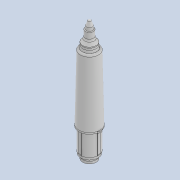
# Autodesk Inventor part: маркер
Saved by Autodesk Inventor 2021.2 (Build 252289000, 289)
## iProperties
Created: 2026-09-22
Part Number: маркер
Material: Типовые
Document SubType Name: Modeling
Designer: ritar
Density: 1 g/cm^3
Appearance: По умолчанию
Author: ritar
Autodesk Inventor part; units mm, degrees
ref_plane "YZ Plane" through (0, 0, 0) normal (1, 0, 0) x (0, 1, 0)
ref_plane "XZ Plane" through (0, 0, 0) normal (0, 1, 0) x (-1, 0, 0)
ref_plane "XY Plane" through (0, 0, 0) normal (0, 0, 1) x (1, 0, 0)
sketch "Эскиз1" plane through (0, 0, 0) normal (0, 0, 1) x (1, 0, 0)
  line L0 (0, 0) -> (-11.15, 0)
  line L1 (-11.15, 0) -> (-9.75, 67.9856)
  line L2 (-9.75, 67.9856) -> (0, 67.9856)
  line L3 (0, 67.9856) -> (0, 0)
  line L4 (0, 67.9856) -> (0, 70.4856)
  line L5 (-9.75, 67.9856) -> (-9.6985, 70.4856)
  line L6 (0, 70.4856) -> (-9.6985, 70.4856)
  dimension "d0" = 11.15
  dimension "d1" = 9.75
  dimension "d2" = 68
  dimension "d3" = 2.5
  constraints: 14 end point, 3 horizontal, 1 collinear, 1 perpendicular, 1 point on line
  measures "d0" distance of L0.start L0.end
  measures "d1" distance of L1.end L2.end
  measures "d2" distance of L0.end L1.end
  measures "d3" distance of L2.end L4.end
revolve "Вращение1" add sketch "Эскиз1" angle 360 about axis through (0, 67.9856, 0) along (0, -1, 0)
fillet "Сопряжение1" radius 2 1 edges at (9.6985, 70.4856, 0)
sketch "Эскиз2" plane through (0, 0, 0) normal (0, 0, 1) x (1, 0, 0)
  line L0 (-7.7393, 70.4856) -> (7.7393, 70.4856) projected
  line L1 (0, 70.4856) -> (0, 72.9856)
  line L2 (0, 72.9856) -> (-7.2, 72.9856)
  line L3 (-7.2, 72.9856) -> (-7.7, 70.4856)
  line L4 (0, 72.9856) -> (-7.2, 72.9856)
  line L5 (-7.2, 72.9856) -> (-7.2, 74.9856)
  line L6 (-7.2, 74.9856) -> (0, 74.9856)
  line L7 (0, 74.9856) -> (0, 72.9856)
  line L8 (-7.2, 75.9856) -> (0, 75.9856)
  line L9 (0, 75.9856) -> (0, 74.9856)
  arc A0 (-7.2, 75.9856) -> (-7.2, 74.9856) centre (-4.725, 75.4856) ccw
  line L10 (-7.2, 75.9856) -> (-4.3, 79.9856)
  line L11 (-4.3, 79.9856) -> (0, 79.9856)
  line L12 (0, 79.9856) -> (0, 75.9856)
  line L13 (-4.3, 79.9856) -> (0, 79.9856)
  line L14 (0, 79.9856) -> (0, 87.4856)
  line L15 (0, 87.4856) -> (-4.3, 87.4856)
  line L16 (-4.3, 87.4856) -> (-4.3, 79.9856)
  arc A1 (-5.025, 78.9856) -> (-4.3, 81.2207) centre (-8.108, 81.2207) ccw
  line L17 (0, 87.4856) -> (-3.075, 87.4856)
  line L18 (-3.075, 87.4856) -> (-3.075, 90.9856)
  line L19 (-3.075, 90.9856) -> (0, 90.9856)
  line L20 (0, 90.9856) -> (0, 87.4856)
  line L21 (-3.075, 90.9856) -> (-1.5669, 95.3677)
  arc A2 (0, 96.4856) -> (-1.5669, 95.3677) centre (0, 94.8285) ccw
  line L22 (0, 90.9856) -> (0, 96.4856)
  point P0 (0, 0)
  point P1 (-7.25, 75.4856)
  point P2 (-3.075, 87.4856)
  dimension "d6" = 7.2
  dimension "d7" = 7.7
  dimension "d8" = 2.5
  dimension "d9" = 2
  dimension "d10" = 1
  dimension "d12" = 0.05
  dimension "d13" = 4.3
  dimension "d14" = 4
  dimension "d15" = 17
  dimension "d16" = 1
  dimension "d17" = 1.2352
  dimension "d18" = 3.075
  dimension "d19" = 3.5
  dimension "d20" = 5.5
  constraints: 44 end point, 7 parallel, 7 point on circle, 5 horizontal, 5 perpendicular, 3 centre point, 3 point on line, 3 tangent, 3 vertical alignment, 2 vertical, 1 midpoint
  measures "d6" distance of L2.end L1.end
  measures "d7" distance from line of L3.end L1
  measures "d8" distance of L1.start L1.end
  measures "d9" distance of L6.end L1.end
  measures "d10" distance of L8.end L6.end
  measures "d12" horizontal distance of L5.end point (-7.25, 75.486)
  measures "d13" distance of L10.end L11.end
  measures "d14" distance of L11.end L8.end
  measures "d15" distance between parallel lines of L0 L15
  measures "d16" distance from line of L11 A1.start
  measures "d17" vertical distance of L11.end A1.end
  measures "d18" distance of L18.end L19.end
  measures "d19" distance of L17.end L18.end
  measures "d20" distance of L19.end L22.end
revolve "Вращение2" add sketch "Эскиз2" angle 360 about axis through (0, 79.9856, 0) along (0, 1, 0)
sketch "Эскиз3" plane through (0, 0, 0) normal (0, -1, 0) x (1, 0, 0)
  circle A0 centre (0, 0) radius 11.15 projected
extrude "Выдавливание1" add sketch "Эскиз3" along normal blind 1.5
sketch "Эскиз4" plane through (0, 0, 0) normal (0, 0, 1) x (1, 0, 0)
  line L0 (-11.15, -1.5) -> (11.15, -1.5) projected
  line L1 (0, -1.5) -> (0, -24)
  line L2 (0, -24) -> (-9.6, -24)
  line L3 (-9.6, -24) -> (-9.75, -1.5)
  line L4 (-9.75, -1.5) -> (0, -1.5)
  line L5 (-9.6, -24) -> (-9.5833, -26.5)
  line L6 (-9.5833, -26.5) -> (0, -26.5)
  line L7 (0, -26.5) -> (0, -24)
  arc A0 (-9.6, -24) -> (-9.2661, -26.5) centre (0.4274, -23.9332) ccw
  line L8 (0, -26.5) -> (-7.4, -26.5)
  line L9 (-7.4, -26.5) -> (-7.4, -29)
  line L10 (-7.4, -29) -> (0, -29)
  line L11 (0, -29) -> (0, -26.5)
  line L12 (0, -29) -> (-7.2, -29)
  line L13 (-7.2, -29) -> (-7.2, -31.5)
  line L14 (-7.2, -31.5) -> (0, -31.5)
  line L15 (0, -31.5) -> (0, -29)
  line L16 (-7.2, -31.5) -> (0, -33)
  line L17 (0, -31.5) -> (0, -33)
  point P0 (0, 0)
  point P1 (-9.75, -1.5)
  dimension "d24" = 9.6
  dimension "d25" = 9.75
  dimension "d26" = 22.5
  dimension "d27" = 2.5
  dimension "d28" = 2.5
  dimension "d29" = 7.4
  dimension "d30" = 2.5
  dimension "d31" = 7.2
  dimension "d32" = 1.5
  constraints: 34 end point, 5 parallel, 4 perpendicular, 3 horizontal, 2 point on circle, 2 vertical, 1 centre point, 1 collinear, 1 midpoint, 1 point on line, 1 tangent
  measures "d24" distance of L1.end L2.end
  measures "d25" distance from line of L1 L3.end
  measures "d26" distance of L1.start L1.end
  measures "d27" distance of L6.end L1.end
  measures "d28" distance of L10.end L6.end
  measures "d29" distance of L9.end L10.end
  measures "d30" distance of L14.end L10.end
  measures "d31" distance of L13.end L14.end
  measures "d32" distance of L14.end L16.end
revolve "Вращение3" add sketch "Эскиз4" angle 360 about axis through (0, -29, 0) along (0, 1, 0) contours L0 L1 L2 L3 | L2 L7 L6 A0 | L11 L10 L9 L6 | L15 L14 L13 L10 | L17 L16 L14
sketch "Эскиз5" plane through (0, -1.5, 0) normal (0, -1, 0) x (1, 0, 0)
  circle A0 centre (0, 0) radius 11.15 projected
  circle A1 centre (9.346, 0) radius 3
  circle A2 centre (0, 0) radius 11.15 projected
  point P0 (0, 0)
  point P1 (10.8426, -2.6)
  point P2 (10.8426, 2.6)
  point P3 (10.8426, -2.6)
  dimension "d48" = 5.2
  dimension "d50" = 6
  dimension "d51" = 2.6
  constraints: 2 point on circle, 1 centre point, 4 other
  measures "d48" distance of A1.start A1.end
  measures "d50" diameter of A1
  measures "d51" vertical distance of A1.end A1.centre
sketch "Эскиз6" plane through (0, -1.5, 0) normal (0, -1, 0) x (1, 0, 0)
  line L0 (10.35, 1.45) -> (8.1099, 1.45)
  line L1 (8.1099, 1.45) -> (8.1099, -1.45)
  line L2 (8.1099, -1.45) -> (10.35, -1.45)
  line L3 (10.35, -1.45) -> (10.35, 1.45)
  circle A0 centre (0, 0) radius 9.75 projected
  point P0 (0, 0)
  dimension "d37" = 2.9
  dimension "d38" = 1.45
  dimension "d39" = 0.6
  constraints: 8 end point, 2 parallel, 1 horizontal, 1 perpendicular
  measures "d37" distance of L2.end L0.start
  measures "d38" distance from line of point (0, 0) L0
  measures "d39" distance edge to line of A0 L3
extrude "Выдавливание3" add sketch "Эскиз6" along normal blind 22.5 contours L3 L2 A0 L0 | A0 L2 L1 L0 picked at (8.6566, 0)
chamfer "Фаска1" distance 0.6 distance2 1.6 1 edges at (10.35, -24, 0) measured on face at (10.0959, -24, 0.1617)
pattern_circular "Круговой массив1" count 4 over 360 about axis through (0, -10, 0) along (0, 1, 0) of "Выдавливание3", "Фаска1"
extrude "Выдавливание4" add sketch "Эскиз5" against normal blind 1.5 contours A0 A1 picked at (11.5153, -0.4994)
